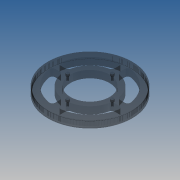
# Autodesk Inventor part: 235 drive pulley
Saved by Autodesk Inventor 2013 (Build 170138000, 138)
## iProperties
Created: 2017-03-15
Part Number: 235 drive pulley
Material: Generic
Document SubType Name: Modeling
Designer: employee
Density: 1 g/cm^3
Author: employee
Autodesk Inventor part; units mm, degrees
ref_plane "YZ Plane" through (0, 0, 0) normal (1, 0, 0) x (0, 1, 0)
ref_plane "XZ Plane" through (0, 0, 0) normal (0, 1, 0) x (-1, 0, 0)
ref_plane "XY Plane" through (0, 0, 0) normal (0, 0, 1) x (1, 0, 0)
sketch "Sketch11" plane through (0, 0, 0) normal (0, 0, 1) x (1, 0, 0)
  circle A0 centre (0, 0) radius 74.5488
  dimension "d78" = 149.0976
  constraints: 1 centre point, 1 coincident
  measures "d78" diameter of A0
extrude "Extrusion11" add sketch "Sketch11" along normal mid plane 8
sketch "Sketch12" plane through (0, 0, -4) normal (0, 0, -1) x (-1, 0, 0)
  circle A0 centre (0, 0) radius 74.5488 projected
  circle A1 centre (0, 74.5488) radius 0.795
  dimension "d82" = 1.59
  constraints: 2 vertical alignment, 1 centre point, 1 other
  measures "d82" diameter of A1
extrude "Extrusion12" cut sketch "Sketch12" against normal through all contours A1 A0 | A0 A1 picked at (-0.0318, 74.2854) picked at (0.0313, 74.8116)
pattern_circular "Circular Pattern4" count 235 over 360 about axis through (0, 0, 0) along (0, 0, 1) of "Extrusion12"
sketch "Sketch13" plane through (0, 0, 4) normal (0, 0, 1) x (1, 0, 0)
  arc A0 (-55.4879, 49.7858) -> (-55.7563, 49.4849) centre (0, 0) ccw projected
  arc A1 (3.1904, 74.4805) -> (2.7876, 74.4967) centre (0, 0) ccw projected
  circle A2 centre (0, 0) radius 75.5488
  dimension "d96" = 1
  constraints: 1 centre point, 1 coincident
  measures "d96" radial gap between concentric circles of A0 A2
extrude "Extrusion16" add sketch "Sketch13" along normal blind 2.5
mirror "Mirror2" about plane through (0, 0, 0) normal (0, 0, 1) of "Extrusion16"
chamfer "Chamfer3" distance 1 angle 45 2 edges at (-75.5488, 0, -4) (-75.5488, 0, 4)
sketch "Sketch14" plane through (0, 0, -6.5) normal (0, 0, -1) x (-1, 0, 0)
  circle A0 centre (0, 0) radius 75.5488 projected
  circle A1 centre (0, 0) radius 35
  circle A2 centre (0, 0) radius 45
  circle A3 centre (0, 0) radius 63.5488
  dimension "d102" = 12
  dimension "d103" = 70
  dimension "d104" = 10
  constraints: 3 centre point, 3 coincident
  measures "d102" radial gap between concentric circles of A0 A3
  measures "d103" diameter of A1
  measures "d104" radial gap between concentric circles of A2 A1
extrude "Extrusion17" cut sketch "Sketch14" against normal through all contours A1 | A3
sketch "Sketch8" plane through (0, 0, -6.5) normal (0, 0, -1) x (-1, 0, 0)
  circle A0 centre (0, 0) radius 45
  circle A1 centre (0, 0) radius 75.5488
  circle A2 centre (0, 0) radius 63.5488
  line L0 (-5, 63.5488) -> (5, 63.5488)
  line L1 (5, 63.5488) -> (5, 44.7214)
  line L2 (5, 44.7214) -> (-5, 44.7214)
  line L3 (-5, 44.7214) -> (-5, 63.5488)
  circle A3 centre (0, 0) radius 45 projected
  circle A4 centre (0, 0) radius 63.5488 projected
  circle A5 centre (0, 0) radius 75.5488 projected
  dimension "d60" = 10
  constraints: 8 end point, 3 centre point, 3 coincident, 3 concentric, 2 parallel, 2 point on circle, 1 horizontal, 1 perpendicular, 1 tangent
  measures "d60" distance between parallel lines of L1 L3
extrude "Extrusion8" add sketch "Sketch8" against normal up to surface (13 mm away) contours A0 L3 A2 L1 | A2 L0 L1 | L3 L0 A2 picked at (0, 51.1623)
pattern_circular "Circular Pattern5" count 4 over 360 about axis through (0, 0, -6.5) along (0, 0, 1) of "Extrusion8"
fillet "Fillet2" radius 5 16 edges at (5, -63.3518, 0) (5, -44.7214, 0) (63.3518, -5, 0) (44.7214, -5, 0) (44.7214, 5, 0) (63.3518, 5, 0) (5, 44.7214, 0) (5, 63.3518, 0) (-44.7214, 5, 0) (-63.3518, 5, 0) (-63.3518, -5, 0) (-44.7214, -5, 0) (-5, -44.7214, 0) (-5, -63.3518, 0) (-5, 44.7214, 0) (-5, 63.3518, 0)
sketch "Sketch9" plane through (0, 0, 6.5) normal (0, 0, 1) x (1, 0, 0)
  circle A0 centre (-40, 0) radius 1.75
  arc A1 (44.0908, 9) -> (9, 44.0908) centre (0, 0) ccw projected
  arc A2 (62.615, 10.854) -> (10.854, 62.615) centre (0, 0) ccw projected
  dimension "d69" = 3.5
  dimension "d111" = 40
  constraints: 1 centre point, 1 horizontal alignment
  measures "d69" diameter of A0
  measures "d111" distance of A0.centre A2.centre
extrude "Extrusion18" cut sketch "Sketch9" against normal through all
sketch "Sketch15" plane through (0, 0, 6.5) normal (0, 0, 1) x (1, 0, 0)
  circle A0 centre (-40, 0) radius 1.75 projected
  line L0 (-40, 3.1754) -> (-37.25, 1.5877)
  line L1 (-37.25, 1.5877) -> (-37.25, -1.5877)
  line L2 (-37.25, -1.5877) -> (-40, -3.1754)
  line L3 (-40, -3.1754) -> (-42.75, -1.5877)
  line L4 (-42.75, -1.5877) -> (-42.75, 1.5877)
  line L5 (-42.75, 1.5877) -> (-40, 3.1754)
  dimension "d114" = 5.5
  constraints: 12 end point, 1 coincident, 1 vertical, 13 other
  measures "d114" distance between parallel lines of L4 L1
extrude "Extrusion19" cut sketch "Sketch15" against normal blind 4
pattern_circular "Circular Pattern6" count 4 over 360 about axis through (0, 0, -6.5) along (0, 0, 1) of "Extrusion19", "Extrusion18"
equation "\"errode\" = 0.1"
body "Solid1"
body "Solid2"
